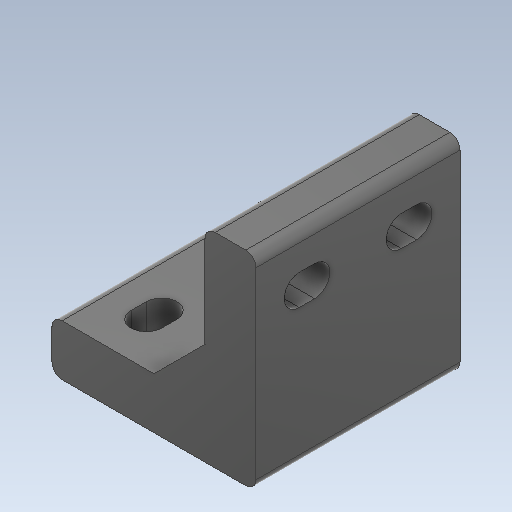
# Autodesk Inventor part: 0008-10-022 Suport L
Saved by Autodesk Inventor 2020 (Build 240168000, 168)
## iProperties
Created: 2021-03-06
Part Number: 0008-10-022 Suport L
Material: ABS Plastic
Document SubType Name: Modeling
Designer: Iulian Bors
Density: 1.06 g/cm^3
Appearance: Smooth - White
Mass: 29.656 g
Surface Area: 81.0921 cm^2
Volume: 27.9773 cm^3
Description: Suport L
Author: Iulian Bors
Subject: 023
Autodesk Inventor part; units mm, degrees
ref_plane "YZ Plane" through (0, 0, 0) normal (1, 0, 0) x (0, 1, 0)
ref_plane "XZ Plane" through (0, 0, 0) normal (0, 1, 0) x (-1, 0, 0)
ref_plane "XY Plane" through (0, 0, 0) normal (0, 0, 1) x (1, 0, 0)
sketch "Sketch1" plane through (0, 0, 0) normal (0, 0, 1) x (1, 0, 0)
  line L0 (-40, 5) -> (0, 5)
  line L1 (0, 5) -> (0, -5)
  line L2 (0, -5) -> (-40, -5)
  line L3 (-40, -5) -> (-40, 5)
  line L4 (-10, 35) -> (0, 35)
  line L5 (0, 35) -> (0, 5)
  line L6 (0, 5) -> (-10, 5)
  line L7 (-10, 5) -> (-10, 35)
  point P0 (0, 0)
  point P1 (0, 5)
  dimension "d0" = 10
  dimension "d1" = 40
  dimension "d2" = 40
  constraints: 16 end point, 4 parallel, 3 perpendicular, 2 horizontal, 1 collinear, 1 midpoint, 1 point on line
  measures "d0" distance of L2.end L0.start
  measures "d1" distance of L1.end L2.end
  measures "d2" distance between parallel lines of L2 L4
extrude "Extrusion1" add sketch "Sketch1" along normal blind 40
sketch "Sketch2" plane through (-10, 5, 0) normal (-1, 0, 0) x (0, 0, 1)
  line L0 (8.5, 20) -> (11.5, 20) construction
  line L1 (8.5, 17) -> (11.5, 17)
  line L2 (11.5, 23) -> (8.5, 23)
  arc A0 (8.5, 23) -> (8.5, 17) centre (8.5, 20) ccw
  arc A1 (11.5, 17) -> (11.5, 23) centre (11.5, 20) ccw
  line L3 (0, 30) -> (0, 0) projected
  line L4 (0, 30) -> (40, 30) projected
  line L5 (20, 21.547) -> (20, 15) construction
  line L6 (31.5, 20) -> (28.5, 20) construction
  line L7 (31.5, 17) -> (28.5, 17)
  line L8 (28.5, 23) -> (31.5, 23)
  arc A2 (31.5, 17) -> (31.5, 23) centre (31.5, 20) ccw
  arc A3 (28.5, 23) -> (28.5, 17) centre (28.5, 20) ccw
  point P0 (0, -5)
  point P1 (10, 20)
  point P2 (20, 18.2735)
  point P3 (20, 30)
  point P4 (30, 20)
  dimension "d5" = 6
  dimension "d6" = 3
  dimension "d7" = 10
  dimension "d8" = 10
  constraints: 18 end point, 8 point on circle, 7 symmetric about line, 4 centre point, 4 tangent, 3 midpoint, 1 horizontal, 1 parallel, 1 vertical, 1 vertical alignment, 2 other
  measures "d5" diameter of A1
  measures "d6" distance of L0.start L0.end
  measures "d7" distance from line of L3 point (10, 20)
  measures "d8" distance between parallel lines of L0 L4
extrude "Extrusion2" cut sketch "Sketch2" against normal through all
sketch "Sketch3" plane through (-40, 5, 0) normal (0, 1, 0) x (1, 0, 0)
  line L0 (10, -8.5) -> (10, -11.5) construction
  line L1 (7, -8.5) -> (7, -11.5)
  line L2 (13, -11.5) -> (13, -8.5)
  arc A0 (13, -8.5) -> (7, -8.5) centre (10, -8.5) ccw
  arc A1 (7, -11.5) -> (13, -11.5) centre (10, -11.5) ccw
  line L3 (30, 0) -> (0, 0) projected
  line L4 (0, 0) -> (0, -40) projected
  line L5 (15.2557, -20) -> (9.287, -20) construction
  line L6 (10, -31.5) -> (10, -28.5) construction
  line L7 (7, -31.5) -> (7, -28.5)
  line L8 (13, -28.5) -> (13, -31.5)
  arc A2 (7, -31.5) -> (13, -31.5) centre (10, -31.5) ccw
  arc A3 (13, -28.5) -> (7, -28.5) centre (10, -28.5) ccw
  point P0 (40, 0)
  point P1 (10, -10)
  point P2 (12.2713, -20)
  point P3 (0, -20)
  point P4 (10, -30)
  dimension "d11" = 3
  dimension "d12" = 6
  dimension "d13" = 10
  dimension "d14" = 10
  constraints: 18 end point, 8 point on circle, 7 symmetric about line, 4 centre point, 4 tangent, 3 midpoint, 1 horizontal, 1 horizontal alignment, 1 parallel, 1 vertical, 2 other
  measures "d11" distance of L0.start L0.end
  measures "d12" distance between parallel lines of L1 L2
  measures "d13" distance from line of L3 point (10, -10)
  measures "d14" distance between parallel lines of L4 L0
extrude "Extrusion3" cut sketch "Sketch3" against normal through all
chamfer "Chamfer1" distance 10 angle 45 1 edges at (-10, 5, 20)
fillet "Fillet1" radius 2 5 edges at (-10, 35, 20) (0, 35, 20) (0, -5, 20) (-40, -5, 20) (-40, 5, 20)
equation "\"d2\" = d1"
body "Solid1"
